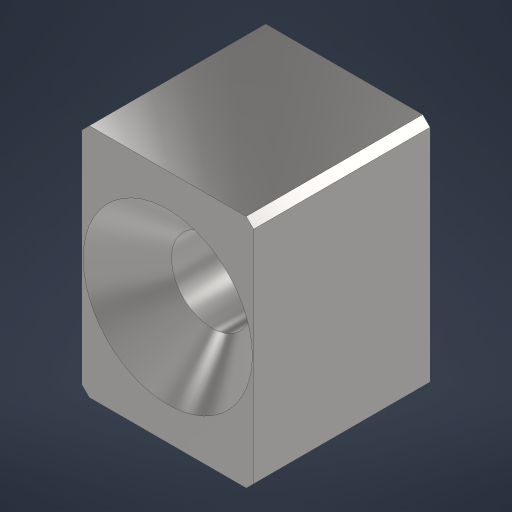
# Autodesk Inventor part: TH1-002
Saved by Autodesk Inventor 2024.3 (Build 283343000, 343)
## iProperties
Created: 2024-01-14
Part Number: TH1-002
Material: Steel, Mild
Document SubType Name: Modeling
Designer: fablabadmin
Density: 7.85 g/cm^3
Appearance: Semi-Polished
Stock Number: SS1672
Description: Holder tooth
Author: Benjamin Solar
Revision Number: 2
Autodesk Inventor part; units mm, degrees
ref_plane "YZ Plane" through (0, 0, 0) normal (1, 0, 0) x (0, 1, 0)
ref_plane "XZ Plane" through (0, 0, 0) normal (0, 1, 0) x (-1, 0, 0)
ref_plane "XY Plane" through (0, 0, 0) normal (0, 0, 1) x (1, 0, 0)
sketch "Sketch1" plane through (0, 0, 0) normal (0, 0, 1) x (1, 0, 0)
  line L0 (23.825, 8.05) -> (23.825, -8.05) construction
  line L1 (37, 8) -> (31.3548, 8) construction
  line L2 (31.3548, -8) -> (37, -8) construction
  line L3 (37, 8) -> (23.825, 8) construction
  line L4 (23.825, 8) -> (23.825, -8) construction
  line L5 (23.825, -8) -> (37, -8) construction
  line L6 (37, -8) -> (37, 8) construction
  circle A0 centre (30.6625, 0) radius 2.067 construction
  line L7 (36.5, -8) -> (24.825, -8)
  line L8 (24.825, -8) -> (24.825, 8)
  line L9 (24.825, 8) -> (36.5, 8)
  line L10 (36.5, 8) -> (36.5, -8)
  line L11 (36.5, -8) -> (24.825, 8) construction
  line L12 (24.825, -8) -> (36.5, 8) construction
  point P0 (0, 0)
  dimension "d0" = 1
  dimension "d1" = 0
  dimension "d11" = 11.675
  dimension "d12" = 16
  constraints: 20 end point, 4 parallel, 2 horizontal, 2 midpoint, 2 perpendicular, 2 point on line
  measures "d0" distance between parallel lines of L8 L0
  measures "d1" distance between parallel lines of L1 L9
  measures "d11" distance between parallel lines of L10 L8
  measures "d12" distance between parallel lines of L9 L7
extrude "Extrusion1" add sketch "Sketch1" along normal blind 12
sketch "Sketch2" plane through (0, 0, 12) normal (0, 0, 1) x (1, 0, 0)
  point P0 (0, 0)
  point P1 (30.6625, 0)
hole "Hole1" at (30.6625, 0, 12) direction (0, 0, -1) diameter 5.5 end through all countersink diameter 11.5 countersink angle 90 clearance for "Countersunk Flat Head Screw ISO 2009/7046" size "M5" standard "ISO"
chamfer "Chamfer1" distance 0.5 angle 45 4 edges at (24.825, -8, 6) (24.825, 8, 6) (36.5, 8, 6) (36.5, -8, 6)
chamfer "Chamfer2" distance 0.5 angle 45 1 edges at (30.6625, 2.75, 0)
body "Solid1"
